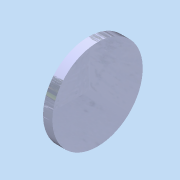
# Autodesk Inventor part: 카메라 창
Saved by Autodesk Inventor 2020 (Build 240168000, 168)
## iProperties
Created: 2020-05-05
Part Number: 카메라 창
Material: 일반
Document SubType Name: Modeling
Designer: sbahn
Density: 1 g/cm^3
Appearance: 선명
Author: sbahn
Autodesk Inventor part; units mm, degrees
ref_plane "YZ Plane" through (0, 0, 0) normal (1, 0, 0) x (0, 1, 0)
ref_plane "XZ Plane" through (0, 0, 0) normal (0, 1, 0) x (-1, 0, 0)
ref_plane "XY Plane" through (0, 0, 0) normal (0, 0, 1) x (1, 0, 0)
sketch "스케치1" plane through (0, 0, 0) normal (0, 0, 1) x (1, 0, 0)
  line L0 (0, 0) -> (8.9929, 0)
  line L1 (1.6697, 5) -> (1.6697, -5) projected
  line L2 (1.6697, 0) -> (1.6697, -5)
  line L3 (1.6697, -5) -> (0.6351, -5)
  line L4 (1.6697, -5) -> (0.6351, -5)
  arc A0 (0, 0) -> (0.6351, -5) centre (18.0758, -0.2444) ccw
  point P0 (1.6697, 0)
  constraints: 8 end point, 3 horizontal, 2 point on circle, 1 centre point, 1 collinear, 1 midpoint, 1 other
revolve "회전1" add sketch "스케치1" angle 360 about axis through (0, 0, 0) along (1, 0, 0)
